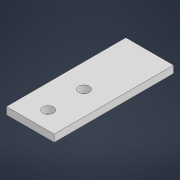
# Autodesk Inventor part: Endstop Mounting Plate
Saved by Autodesk Inventor 2022 (Build 260153000, 153)
## iProperties
Created: 2023-06-23
Part Number: Endstop Mounting Plate
Material: Generic
Document SubType Name: Modeling
Designer: Ryan Mitcham
Density: 1 g/cm^3
Appearance: Default
Author: Ryan Mitcham
Autodesk Inventor part; units mm, degrees
ref_plane "YZ Plane" through (0, 0, 0) normal (1, 0, 0) x (0, 1, 0)
ref_plane "XZ Plane" through (0, 0, 0) normal (0, 1, 0) x (-1, 0, 0)
ref_plane "XY Plane" through (0, 0, 0) normal (0, 0, 1) x (1, 0, 0)
sketch "Sketch1" plane through (0, 0, 0) normal (0, 1, 0) x (-1, 0, 0)
  line L0 (10, 25) -> (-10, 25)
  line L1 (-10, 25) -> (-10, -25)
  line L2 (-10, -25) -> (10, -25)
  line L3 (10, -25) -> (10, 25)
  point P0 (0, 0)
  point P1 (0, -25)
  point P2 (10, 0)
  dimension "d0" = 20
  dimension "d1" = 50
  constraints: 8 end point, 2 midpoint, 2 parallel, 1 horizontal, 1 horizontal alignment, 1 perpendicular, 1 vertical alignment
  measures "d0" distance of L2.end L1.end
  measures "d1" distance of L2.end L0.start
extrude "Extrusion1" add sketch "Sketch1" along normal blind 3
sketch "Sketch2" plane through (0, 3, 0) normal (0, 1, 0) x (1, 0, 0)
  line L0 (-10, -25) -> (10, -25) projected
  point P0 (0, 0)
  point P1 (0, -17.5)
  point P2 (0, -2.5)
  dimension "d4" = 15
  dimension "d6" = 7.5
  constraints: 2 vertical alignment
  measures "d4" distance of point (0, -17.5) point (0, -2.5)
  measures "d6" distance from line of L0 point (0, -17.5)
hole "Hole1" at (0, 3, 17.5) at (0, 3, 2.5) direction (0, -1, 0) diameter 4.5 end through all
body "Solid1"
